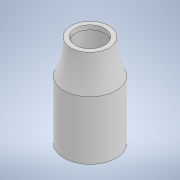
# Autodesk Inventor part: 10mm Nozzle
Saved by Autodesk Inventor 2022 (Build 260153000, 153)
## iProperties
Created: 2023-01-19
Part Number: 10mm Nozzle
Material: Generic
Document SubType Name: Modeling
Designer: ASUS
Density: 1 g/cm^3
Appearance: Default
Author: ASUS
Autodesk Inventor part; units mm, degrees
ref_plane "YZ Plane" through (0, 0, 0) normal (1, 0, 0) x (0, 1, 0)
ref_plane "XZ Plane" through (0, 0, 0) normal (0, 1, 0) x (-1, 0, 0)
ref_plane "XY Plane" through (0, 0, 0) normal (0, 0, 1) x (1, 0, 0)
sketch "Sketch1" plane through (0, 0, 0) normal (0, 1, 0) x (-1, 0, 0)
  circle A0 centre (0, 0) radius 7.5
  circle A1 centre (0, 0) radius 8.875
  dimension "d0" = 15
  dimension "d1" = 17.75
  constraints: 2 centre point, 2 coincident
  measures "d0" diameter of A0
  measures "d1" diameter of A1
extrude "Extrusion1" add sketch "Sketch1" along normal blind 20
sketch "Sketch2" plane through (0, 0, 0) normal (1, 0, 0) x (0, 1, 0)
  line L0 (30, 0) -> (30, -5)
  line L1 (20, 7.5) -> (20, -7.5) projected
  arc A0 (30, -5) -> (20, -7.5) centre (30, -26.25) ccw
  line L2 (30, -5) -> (22.0069, -5) construction
  line L3 (20, -8.875) -> (20, 8.875) projected
  arc A1 (31.5, -6.5) -> (20, -8.875) centre (31.5, -35.5296) ccw
  line L4 (31.5, -6.5) -> (25.6327, -6.5) construction
  line L5 (31.5, 0) -> (31.5, -6.5) construction
  line L6 (30, -5) -> (31.5, -5)
  line L7 (31.5, -5) -> (31.5, -6.5)
  line L8 (20, 0) -> (33.2295, 0)
  point P0 (0, 0)
  dimension "d4" = 5
  dimension "d5" = 10
  dimension "d6" = 0
  dimension "d8" = 1.5
  constraints: 14 end point, 4 point on circle, 3 horizontal, 2 centre point, 2 tangent, 2 vertical, 1 midpoint, 1 perpendicular, 1 point on line
  measures "d4" distance of L0.start L0.end
  measures "d5" distance between parallel lines of L1 L0
  measures "d6" vertical distance of point (0, 0) L0.start
  measures "d8" horizontal distance of L0.end L4.start
revolve "Revolution1" add sketch "Sketch2" angle 360 about axis through (0, 20, 0) along (0, 1, 0) contours L6 L7 A1 L3 A0
body "Solid1"
